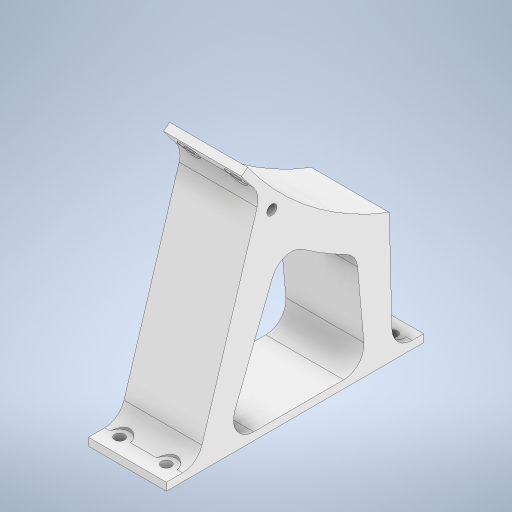
# Autodesk Inventor part: Fuß_Rohr_Innen_1
Saved by Autodesk Inventor 2023 (Build 270158000, 158)
## iProperties
Created: 2023-01-04
Part Number: Fuß_Rohr_Innen_1
Material: Generisch
Document SubType Name: Modeling
Designer: trist
Density: 1 g/cm^3
Appearance: Weiß
Author: trist
Autodesk Inventor part; units mm, degrees
ref_plane "XZ Plane" through (0, 0, 0) normal (0, 1, 0) x (-1, 0, 0)
ref_plane "XY Plane" through (0, 0, 0) normal (0, 0, 1) x (1, 0, 0)
sketch "Skizze1" plane through (0, 0, 0) normal (1, 0, 0) x (0, 1, 0)
  circle A0 centre (0, 0) radius 250 construction
  line L0 (0, 350) -> (0, -350) projected
  arc A1 (-116.1406, 162.8231) -> (-186.5905, 72) centre (0, 0) ccw
  line L1 (-270, 50) -> (-270, 215)
  line L2 (-374, 0) -> (354, 0) projected
  line L3 (-265, 178) -> (-265, 87)
  line L4 (-270, 215) -> (-265, 215)
  line L5 (-265, 215) -> (-265, 195)
  line L6 (0, 0) -> (-116.1406, 162.8231) construction
  line L7 (-116.1406, 162.8231) -> (-119.0441, 166.8937)
  arc A2 (-119.0441, 166.8937) -> (-134.5099, 154.7) centre (0, 0) ccw
  line L8 (-265, 195) -> (-134.5099, 154.7)
  line L9 (-265, 178) -> (-169.1257, 140.7)
  arc A3 (-169.1257, 140.7) -> (-199.3765, 93) centre (0, 0) ccw
  line L10 (-186.5905, 72) -> (-265, 70)
  line L11 (-265, 87) -> (-199.3765, 93)
  line L12 (-265, 70) -> (-265, 50)
  line L13 (-265, 50) -> (-270, 50)
  dimension "d16" = 500
  dimension "d18" = 200
  dimension "d21" = 270
  dimension "d38" = 5
  dimension "d41" = 5
  dimension "d43" = 20
  dimension "d45" = 17
  dimension "d46" = 17
  dimension "d48" = 215
  dimension "d49" = 20
  dimension "d52" = 21
  dimension "d53" = 14
  dimension "d54" = 220
  dimension "d55" = 50
  dimension "d56" = 72
  dimension "d98" = 140.7
  dimension "d99" = 54.5
  constraints: 24 end point, 6 point on circle, 4 centre point, 3 coincident, 3 vertical, 2 perpendicular, 2 vertical alignment, 1 horizontal, 1 line through centre, 1 midpoint, 1 point on line
  measures "d16" diameter of A0
  measures "d18" radius of A1
  measures "d21" distance between parallel lines of L0 L1
  measures "d38" distance between parallel lines of L1 L3
  measures "d41" distance of L6.end L7.end
  measures "d43" distance of L4.end L5.end
  measures "d45" distance of L5.end L3.start
  measures "d46" distance of L3.end L10.end
  measures "d48" distance from line of L2 L1.end
  measures "d49" distance of L10.end L12.end
  measures "d52" vertical distance of L10.start L11.end
  measures "d53" vertical distance of L9.end L8.end
  measures "d54" radius of A3
  measures "d55" distance from line of L2 L12.end
  measures "d56" distance from line of L2 L10.start
  measures "d98" distance from line of L2 L9.end
  measures "d99" angle of L2 L6
extrude "Extrusion2" add sketch "Skizze1" along normal blind 50
sketch "Skizze2" plane through (0, 0, 0) normal (1, 0, 0) x (0, 1, 0)
  line L0 (0, 0) -> (-147.4318, 147.4318) construction
  line L1 (-182.9181, 0) -> (30.4864, 0) projected
  circle A0 centre (-147.4318, 147.4318) radius 3.2
  dimension "d30" = 45
  dimension "d31" = 208.5
  dimension "d32" = 6.4
  constraints: 2 end point, 1 centre point, 1 coincident
  measures "d30" angle of L1 L0
  measures "d31" distance of L0.start L0.end
  measures "d32" diameter of A0
extrude "Extrusion3" cut sketch "Skizze2" along normal through all
fillet "Rundung1" radius 13 7 edges at (25, -134.5099, 154.7) (25, -265, 195) (25, -265, 70) (25, -265, 178) (25, -169.1257, 140.7) (25, -199.3765, 93) (25, -265, 87)
ref_plane "Arbeitsebene1" through (10, 0, 0) normal (1, 0, 0) x (0, 1, 0)
sketch "Skizze3" plane through (0, -265, 215) normal (0, 1, 0) x (1, 0, 0)
  line L0 (0, 0) -> (50, 0) projected
  line L1 (0, 10.409) -> (0, 0) projected
  line L2 (10, 258) -> (10, -43) projected
  point P0 (0, 215)
  point P1 (10, 10)
  dimension "d57" = 10
  constraints: 1 point on line
  measures "d57" distance from line of L0 point (10, 10)
hole "Bohrung1" at (10, -265, 205) direction (0, -1, 0) diameter 6.4 end through all
sketch "Skizze4" plane through (0, -265, 215) normal (0, 1, 0) x (1, 0, 0)
  arc A0 (6.8262, 10.409) -> (13.1738, 10.409) centre (10, 10) ccw projected
  constraints: 1 coincident
hole "Bohrung2" at (10, -265, 205) direction (0, 1, 0) diameter 13 end through all
sketch "Skizze5" plane through (0, -265, 50) normal (0, 1, 0) x (1, 0, 0)
  line L0 (0, 0) -> (50, 0) projected
  line L1 (0, 0) -> (0, -7.3274) projected
  line L2 (10, 93) -> (10, -208) projected
  point P0 (0, 50)
  point P1 (10, -10)
  dimension "d73" = 10
  constraints: 1 point on line
  measures "d73" distance from line of L0 point (10, -10)
hole "Bohrung3" at (10, -265, 60) direction (0, -1, 0) diameter 6.4 end through all
sketch "Skizze6" plane through (0, -265, 50) normal (0, 1, 0) x (1, 0, 0)
  arc A0 (11.7598, -7.3274) -> (8.2402, -7.3274) centre (10, -10) ccw projected
  point P0 (0, 50)
  constraints: 1 coincident
hole "Bohrung4" at (10, -265, 60) direction (0, 1, 0) diameter 13 end through all
sketch "Skizze7" plane through (10, 0, 0) normal (1, 0, 0) x (0, 1, 0)
  line L0 (0, 0) -> (-158.1005, 198.7596)
  line L1 (0, 238.5115) -> (0, -39.7519) projected
  arc A0 (-116.1406, 162.8231) -> (-186.5905, 72) centre (0, 0) ccw construction
  arc A1 (-119.0441, 166.8937) -> (-129.2489, 159.1217) centre (0, 0) ccw construction
  line L2 (-130.6639, 164.267) -> (-125.577, 168.3134)
  line L3 (-125.577, 168.3134) -> (-122.4644, 164.4004)
  line L4 (-125.0956, 162.4072) -> (-121.9846, 158.4961)
  line L5 (-121.9846, 158.4961) -> (-124.5029, 156.5216)
  line L6 (-125.0956, 162.4072) -> (-122.4644, 164.4004)
  line L7 (-124.5029, 156.5216) -> (-130.6639, 164.267)
  dimension "d90" = 38.5
  dimension "d91" = 6.4
  dimension "d92" = 13
  dimension "d93" = 5
  constraints: 14 end point, 3 point on circle, 2 perpendicular, 2 point on line, 1 collinear, 1 parallel
  measures "d90" angle of L1 L0
  measures "d91" diameter of L4 L0
  measures "d92" diameter of L3 L0
  measures "d93" distance of L2.end L3.end
revolve "Umdrehung1" cut sketch "Skizze7" angle 360 about axis through (10, 0, 0) along (0, -0.6225146, 0.7826082)
pattern_linear "Rechteckige Anordnung1" count 2 spacing 30 along (1, 0, 0) of "Bohrung1", "Bohrung2", "Bohrung3", "Bohrung4", "Umdrehung1"
ref_plane "Arbeitsebene2" through (40, 0, 0) normal (1, 0, 0) x (0, 1, 0)
